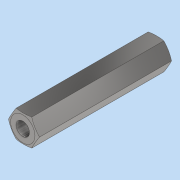
# Autodesk Inventor part: Hex Spacer 20mm
Saved by Autodesk Inventor 2021 (Build 250183000, 183)
## iProperties
Created: 2020-07-05
Part Number: Hex Spacer 20mm
Material: Generisch
Document SubType Name: Modeling
Designer: JochenAlt
Density: 1 g/cm^3
Appearance: Stahl - poliert
Author: JochenAlt
Autodesk Inventor part; units mm, degrees
ref_plane "YZ Plane" through (0, 0, 0) normal (1, 0, 0) x (0, 1, 0)
ref_plane "XZ Plane" through (0, 0, 0) normal (0, 1, 0) x (-1, 0, 0)
ref_plane "XY Plane" through (0, 0, 0) normal (0, 0, 1) x (1, 0, 0)
sketch "Skizze1" plane through (0, 0, 0) normal (0, 0, 1) x (1, 0, 0)
  line L0 (-3.2332, 0) -> (3.2332, 0) construction
  line L1 (0, -2.8) -> (0, 2.8) construction
  circle A0 centre (0, 0) radius 2 construction
  line L2 (1.1547, 2) -> (2.3094, 0)
  line L3 (2.3094, 0) -> (1.1547, -2)
  line L4 (1.1547, -2) -> (-1.1547, -2)
  line L5 (-1.1547, -2) -> (-2.3094, 0)
  line L6 (-2.3094, 0) -> (-1.1547, 2)
  line L7 (-1.1547, 2) -> (1.1547, 2)
  circle A1 centre (0, 0) radius 1
  point P0 (0, 2)
  dimension "d0" = 4
  dimension "d1" = 2
  constraints: 12 end point, 3 coincident, 1 centre point, 1 midpoint, 1 point on line, 1 vertical alignment, 15 other
  measures "d1" diameter of A1
extrude "Extrusion1" add sketch "Skizze1" along normal blind 20
sketch "Skizze2" plane through (0, 0, 0) normal (0, 1, 0) x (-1, 0, 0)
  line L0 (1.1547, 20) -> (-1.1547, 20) projected
  line L1 (-1.1547, 20) -> (-2.3094, 20) projected
  line L2 (2.3094, 20) -> (1.1547, 20) projected
  line L3 (2.3094, 0) -> (1.1547, 0) projected
  line L4 (1.1547, 0) -> (-1.1547, 0) projected
  line L5 (-1.1547, 0) -> (-2.3094, 0) projected
  line L6 (-1.8094, 20) -> (-3.6188, 20)
  line L7 (-3.6188, 20) -> (-3.6188, 19.3414)
  line L8 (-3.6188, 19.3414) -> (-1.8094, 20)
  line L9 (-1.8094, 0) -> (-3.6188, 0.6586)
  line L10 (-3.6188, 0.6586) -> (-3.6188, 0)
  line L11 (-3.6188, 0) -> (-1.8094, 0)
  line L12 (0, -2) -> (0, 12) projected
  point P0 (0, 0)
  dimension "d4" = 20
  dimension "d5" = 0.5
  constraints: 12 end point, 2 equal length, 2 perpendicular, 2 point on line, 1 collinear, 1 vertical
  measures "d4" angle of L6 L8
  measures "d5" distance of L6.start L1.end
revolve "Umdrehung1" cut sketch "Skizze2" angle 360 about axis through (0, 0, -10) along (0, 0, 1)
